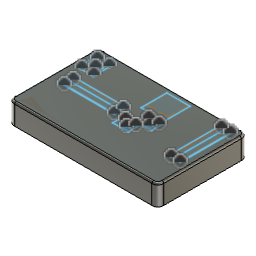
gamepad-g43 (Autodesk Fusion 360 design; units mm, degrees)
Autodesk Fusion 360 part; units mm, degrees
sketch "Sketch1" plane through (0, 0, 0) normal (0, 0, 1) x (1, 0, 0)
  line L0 (-125, 75) -> (125, 75)
  line L1 (125, 75) -> (125, -75)
  line L2 (125, -75) -> (-125, -75)
  line L3 (-125, -75) -> (-125, 75)
  line L4 (-125, 75) -> (125, -75) construction
  dimension "d1" = 250
  dimension "d2" = 150
  constraint horizontal L0
  constraint vertical L1
  constraint horizontal L2
  constraint vertical L3
  constraint midpoint origin L4
  measures "d1" distance of L0.start L0.end
  measures "d2" distance of L0.start L2.end
extrude "Extrude1" add sketch "Sketch1" along normal blind 35
sketch "Sketch3" plane through (0, 0, 0) normal (0, 0, 1) x (1, 0, 0)
  line L0 (-125, -75) -> (125, -75)
  line L1 (125, -75) -> (125, 75)
  line L2 (125, 75) -> (-125, 75)
  line L3 (-125, 75) -> (-125, -75)
  line L4 (-122, 72) -> (122, 72)
  line L5 (122, 72) -> (122, -70)
  line L6 (122, -70) -> (-122, -70)
  line L7 (-122, -70) -> (-122, 72)
  dimension "d7" = 3
  dimension "d8" = 5
  dimension "d9" = 3
  dimension "d10" = 3
  constraint horizontal L4
  constraint vertical L5
  constraint horizontal L6
  constraint vertical L7
  measures "d7" distance of L2 L4
  measures "d8" distance of L0 L6
  measures "d9" distance of L3 L7
  measures "d10" distance of L1 L5
extrude "Extrude2" cut sketch "Sketch3" along normal blind 32 contours L4 L5 L6 L7
fillet "Fillet1" radius 3 4 edges at (125, 0, 35) (0, 75, 35) (-125, 0, 35) (0, -75, 35)
fillet "Fillet1" radius 10 curvature continuous 4 edges at (-125, -75, 17.5) (-125, 75, 17.5) (125, 75, 17.5) (125, -75, 17.5)
fillet "Fillet1" radius 8 curvature continuous 4 edges at (-122, -70, 16) (-122, 72, 16) (122, -70, 16) (122, 72, 16)
sketch "joystick" plane through (0, 0, 35) normal (0, 0, 1) x (-1, 0, 0)
  spline S0 degree 3 poles (-122, 65) (-122, 65.1579) (-122, 65.3156) (-121.9955, 66.0449) (-121.98, 66.6191) (-121.8006, 67.7625) (-121.6245, 68.3289) (-120.9937, 69.5435) (-120.4833, 70.1576) (-119.6074, 70.8914) (-119.3113, 71.0984) (-118.6838, 71.4499) (-118.3524, 71.5936) (-117.5261, 71.8524) (-117.0214, 71.9295) (-116.0107, 72.0014) (-115.5063, 72) (-115, 72) knots -1.149011 -1.149011 -1.149011 -1.149011 -1.101651 -1.101651 -0.930068 -0.930068 -0.754427 -0.754427 -0.519484 -0.519484 -0.411628 -0.411628 -0.303772 -0.303772 -0.151886 -0.151886 0 0 0 0
  line L0 (-122, 65) -> (-122, -65)
  spline S1 degree 3 poles (-115, -72) (-115.1579, -72) (-115.3156, -72) (-116.0449, -71.9955) (-116.6191, -71.98) (-117.7625, -71.8006) (-118.3289, -71.6245) (-119.5435, -70.9937) (-120.1576, -70.4833) (-120.8914, -69.6074) (-121.0984, -69.3113) (-121.4499, -68.6838) (-121.5936, -68.3524) (-121.8524, -67.5261) (-121.9295, -67.0214) (-122.0014, -66.0107) (-122, -65.5063) (-122, -65) knots -1.149011 -1.149011 -1.149011 -1.149011 -1.101651 -1.101651 -0.930068 -0.930068 -0.754427 -0.754427 -0.519484 -0.519484 -0.411628 -0.411628 -0.303772 -0.303772 -0.151886 -0.151886 0 0 0 0
  line L1 (-115, -72) -> (115, -72)
  spline S2 degree 3 poles (122, -65) (122, -65.1579) (122, -65.3156) (121.9955, -66.0449) (121.98, -66.6191) (121.8006, -67.7625) (121.6245, -68.3289) (120.9937, -69.5435) (120.4833, -70.1576) (119.6074, -70.8914) (119.3113, -71.0984) (118.6838, -71.4499) (118.3524, -71.5936) (117.5261, -71.8524) (117.0214, -71.9295) (116.0107, -72.0014) (115.5063, -72) (115, -72) knots -1.149011 -1.149011 -1.149011 -1.149011 -1.101651 -1.101651 -0.930068 -0.930068 -0.754427 -0.754427 -0.519484 -0.519484 -0.411628 -0.411628 -0.303772 -0.303772 -0.151886 -0.151886 0 0 0 0
  line L2 (122, -65) -> (122, 65)
  spline S3 degree 3 poles (115, 72) (115.1579, 72) (115.3156, 72) (116.0449, 71.9955) (116.6191, 71.98) (117.7625, 71.8006) (118.3289, 71.6245) (119.5435, 70.9937) (120.1576, 70.4833) (120.8914, 69.6074) (121.0984, 69.3113) (121.4499, 68.6838) (121.5936, 68.3524) (121.8524, 67.5261) (121.9295, 67.0214) (122.0014, 66.0107) (122, 65.5063) (122, 65) knots -1.149011 -1.149011 -1.149011 -1.149011 -1.101651 -1.101651 -0.930068 -0.930068 -0.754427 -0.754427 -0.519484 -0.519484 -0.411628 -0.411628 -0.303772 -0.303772 -0.151886 -0.151886 0 0 0 0
  line L3 (115, 72) -> (-115, 72)
  line L4 (112.7507, -62.5002) -> (86.7507, -62.5002)
  line L5 (86.7507, -62.5002) -> (86.7507, -28.5002)
  line L6 (86.7507, -28.5002) -> (112.7507, -28.5002)
  line L7 (112.7507, -28.5002) -> (112.7507, -62.5002)
  line L8 (109.7507, -58.5002) -> (89.7507, -58.5002) construction
  line L9 (89.7507, -58.5002) -> (89.7507, -32.5002) construction
  line L10 (89.7507, -32.5002) -> (109.7507, -32.5002) construction
  line L11 (109.7507, -32.5002) -> (109.7507, -58.5002) construction
  line L12 (99.7507, -58.5002) -> (99.7507, -62.5002) construction
  line L13 (89.7507, -45.5002) -> (86.7507, -45.5002) construction
  line L14 (109.7507, -45.5002) -> (112.7507, -45.5002) construction
  circle A0 centre (89.7507, -58.5002) radius 1.5
  circle A1 centre (109.7507, -58.5002) radius 1.5
  circle A2 centre (109.7507, -32.5002) radius 1.5
  circle A3 centre (89.7507, -32.5002) radius 1.5
  line L15 (99.7507, -62.5002) -> (99.7507, -45.5002) construction
  circle A4 centre (99.7507, -45.5002) radius 10
  dimension "d19" = 26
  dimension "d20" = 34
  dimension "d21" = 20
  dimension "d22" = 26
  dimension "d23" = 4
  dimension "d24" = 3
  dimension "d25" = 3
  dimension "d26" = 3
  dimension "d27" = 3
  dimension "d28" = 17
  dimension "d29" = 20
  constraint horizontal L4
  constraint vertical L5
  constraint horizontal L6
  constraint vertical L7
  constraint horizontal L8
  constraint vertical L9
  constraint horizontal L10
  constraint vertical L11
  constraint midpoint L8 L12.start
  constraint midpoint L4 L12.end
  constraint midpoint L9 L13.start
  constraint midpoint L5 L13.end
  constraint midpoint L11 L14.start
  constraint midpoint L7 L14.end
  constraint equal L13 L14
  constraint coincident L8.end L9.start
  constraint coincident L8.start L11.end
  constraint coincident L10.end L11.start
  constraint coincident L9.end L10.start
  constraint perpendicular L4 L15
  constraint coincident L15.end A4.centre
  measures "d19" distance of L4.start L4.end
  measures "d20" distance of L4.start L6.end
  measures "d21" distance of L8.start L8.end
  measures "d22" distance of L8.start L10.end
  measures "d23" distance of L4 L8
  measures "d24" diameter of A0
  measures "d25" diameter of A1
  measures "d26" diameter of A2
  measures "d27" diameter of A3
  measures "d28" distance of L12.end L15.end
  measures "d29" diameter of A4
sketch "keyboard" plane through (0, 0, 35) normal (0, 0, 1) x (-1, 0, 0)
  line L0 (0.8213, -66.0148) -> (-38.1787, -66.0148)
  line L1 (-38.1787, -66.0148) -> (-38.1787, -23.0148)
  line L2 (-38.1787, -23.0148) -> (0.8213, -23.0148)
  line L3 (0.8213, -23.0148) -> (0.8213, -66.0148)
  line L4 (-8.6787, -25.8148) -> (-28.6787, -25.8148) construction
  line L5 (-28.6787, -25.8148) -> (-28.6787, -23.0148) construction
  line L6 (-28.6787, -23.0148) -> (-8.6787, -23.0148) construction
  line L7 (-8.6787, -23.0148) -> (-8.6787, -25.8148) construction
  line L8 (-0.1787, -65.0148) -> (-35.1787, -65.0148) construction
  line L9 (-35.1787, -65.0148) -> (-35.1787, -32.0148) construction
  line L10 (-35.1787, -32.0148) -> (-0.1787, -32.0148) construction
  line L11 (-0.1787, -32.0148) -> (-0.1787, -65.0148) construction
  dimension "d30" = 39
  dimension "d31" = 43
  dimension "d32" = 20
  dimension "d33" = 2.8
  dimension "d34" = 35
  dimension "d35" = 33
  dimension "d36" = 9
  dimension "d37" = 3
  constraint horizontal L0
  constraint vertical L1
  constraint horizontal L2
  constraint vertical L3
  constraint horizontal L4
  constraint vertical L5
  constraint horizontal L6
  constraint vertical L7
  constraint midpoint L2 L6
  constraint horizontal L8
  constraint vertical L9
  constraint horizontal L10
  constraint vertical L11
  measures "d30" distance of L0.start L0.end
  measures "d31" distance of L0.start L2.end
  measures "d32" distance of L4.start L4.end
  measures "d33" distance of L4.start L6.end
  measures "d34" distance of L8.start L8.end
  measures "d35" distance of L8.start L10.end
  measures "d36" distance of L2 L10
  measures "d37" distance of L1 L9
sketch "yaw" plane through (0, 0, 35) normal (0, 0, 1) x (-1, 0, 0)
  line L0 (102.6548, -10.7995) -> (13.6548, -10.7995)
  line L1 (13.6548, -10.7995) -> (13.6548, 9.2005)
  line L2 (13.6548, 9.2005) -> (102.6548, 9.2005)
  line L3 (102.6548, 9.2005) -> (102.6548, -10.7995)
  line L4 (100.1548, -8.2995) -> (16.1548, -8.2995) construction
  line L5 (16.1548, -8.2995) -> (16.1548, 6.7005) construction
  line L6 (16.1548, 6.7005) -> (100.1548, 6.7005) construction
  line L7 (100.1548, 6.7005) -> (100.1548, -8.2995) construction
  line L8 (58.1548, -8.2995) -> (58.1548, -10.7995) construction
  line L9 (58.1548, 6.7005) -> (58.1548, 9.2005) construction
  line L10 (16.1548, -0.7995) -> (13.6548, -0.7995) construction
  line L11 (102.6548, -0.7995) -> (100.1548, -0.7995) construction
  circle A0 centre (100.1548, -8.2995) radius 1.5
  circle A1 centre (100.1548, 6.7005) radius 1.5
  circle A2 centre (16.1548, 6.7005) radius 1.5
  circle A3 centre (16.1548, -8.2995) radius 1.5
  line L12 (96.1548, -1.7995) -> (20.1548, -1.7995)
  line L13 (20.1548, -1.7995) -> (20.1548, 8.2005)
  line L14 (20.1548, 8.2005) -> (96.1548, 8.2005)
  line L15 (96.1548, 8.2005) -> (96.1548, -1.7995)
  line L16 (20.1548, 3.2005) -> (13.6548, 3.2005) construction
  line L17 (96.1548, 3.2005) -> (102.6548, 3.2005) construction
  dimension "d38" = 89
  dimension "d39" = 20
  dimension "d40" = 84
  dimension "d41" = 15
  dimension "d42" = 3
  dimension "d43" = 3
  dimension "d44" = 3
  dimension "d45" = 3
  dimension "d46" = 76
  dimension "d47" = 10
  dimension "d48" = 1
  constraint horizontal L0
  constraint vertical L1
  constraint horizontal L2
  constraint vertical L3
  constraint horizontal L4
  constraint vertical L5
  constraint horizontal L6
  constraint vertical L7
  constraint midpoint L4 L8.start
  constraint midpoint L0 L8.end
  constraint midpoint L6 L9.start
  constraint midpoint L2 L9.end
  constraint midpoint L5 L10.start
  constraint midpoint L1 L10.end
  constraint midpoint L3 L11.start
  constraint midpoint L7 L11.end
  constraint vertical L8
  constraint horizontal L11
  constraint coincident L4.start L7.end
  constraint coincident L6.end L7.start
  constraint coincident L5.end L6.start
  constraint coincident L4.end L5.start
  constraint horizontal L12
  constraint vertical L13
  constraint horizontal L14
  constraint vertical L15
  constraint midpoint L13 L16.start
  constraint coincident L1 L16.end
  constraint perpendicular L1 L16
  constraint midpoint L15 L17.start
  constraint coincident L3 L17.end
  constraint perpendicular L3 L17
  constraint equal L16 L17
  measures "d38" distance of L0.start L0.end
  measures "d39" distance of L0.start L2.end
  measures "d40" distance of L4.start L4.end
  measures "d41" distance of L4.start L6.end
  measures "d42" diameter of A0
  measures "d43" diameter of A1
  measures "d44" diameter of A2
  measures "d45" diameter of A3
  measures "d46" distance of L12.start L12.end
  measures "d47" distance of L12.start L14.end
  measures "d48" distance of L2 L14
sketch "encoder big" plane through (0, 0, 35) normal (0, 0, 1) x (-1, 0, 0)
  line L0 (-14.7711, -17.7922) -> (-40.9711, -17.7922)
  line L1 (-40.9711, -17.7922) -> (-40.9711, 1.4078)
  line L2 (-40.9711, 1.4078) -> (-14.7711, 1.4078)
  line L3 (-14.7711, 1.4078) -> (-14.7711, -17.7922)
  line L4 (-24.1711, -12.1922) -> (-36.5711, -12.1922)
  line L5 (-36.5711, -12.1922) -> (-36.5711, -0.3922)
  line L6 (-36.5711, -0.3922) -> (-24.1711, -0.3922)
  line L7 (-24.1711, -0.3922) -> (-24.1711, -12.1922)
  circle A0 centre (-30.3711, -6.2922) radius 3.4
  line L8 (-24.1711, -0.3922) -> (-36.5711, -12.1922) construction
  line L9 (-19.2711, -15.7922) -> (-36.4711, -15.7922) construction
  circle A1 centre (-19.2711, -15.7922) radius 1.5
  circle A2 centre (-36.4711, -15.7922) radius 1.5
  dimension "d49" = 26.2
  dimension "d50" = 19.2
  dimension "d51" = 12.4
  dimension "d52" = 11.8
  dimension "d53" = 16.8
  dimension "d54" = 17.4
  dimension "d55" = 6.8
  dimension "d57" = 2
  dimension "d58" = 4.5
  dimension "d59" = 4.5
  dimension "d60" = 3
  dimension "d61" = 3
  constraint horizontal L0
  constraint vertical L1
  constraint horizontal L2
  constraint vertical L3
  constraint horizontal L4
  constraint vertical L5
  constraint horizontal L6
  constraint vertical L7
  constraint midpoint A0.centre L8
  constraint parallel L0 L9
  constraint coincident L9.start A1.centre
  constraint coincident L9.end A2.centre
  measures "d49" distance of L0.start L0.end
  measures "d50" distance of L0.start L2.end
  measures "d51" distance of L4.start L4.end
  measures "d52" distance of L4.start L6.end
  measures "d53" distance of L1 L7
  measures "d54" distance of L0 L6
  measures "d55" diameter of A0
  measures "d57" distance of L0 L9
  measures "d58" distance of L3 L9.start
  measures "d59" distance of L1 L9.end
  measures "d60" diameter of A1
  measures "d61" diameter of A2
sketch "encoder small" plane through (0, 0, 35) normal (0, 0, 1) x (-1, 0, 0)
  line L0 (-19.076, 21.1996) -> (-6.676, 21.1996)
  circle A0 centre (-1.776, 5.7996) radius 1.5
  line L1 (2.724, 3.7996) -> (-23.476, 3.7996)
  circle A1 centre (-18.976, 5.7996) radius 1.5
  line L2 (-1.776, 5.7996) -> (-18.976, 5.7996) construction
  line L3 (-6.676, 21.1996) -> (-6.676, 9.3996)
  line L4 (-23.476, 3.7996) -> (-23.476, 22.9996)
  line L5 (-6.676, 21.1996) -> (-19.076, 9.3996) construction
  line L6 (2.724, 22.9996) -> (2.724, 3.7996)
  line L7 (-6.676, 9.3996) -> (-19.076, 9.3996)
  line L8 (-23.476, 22.9996) -> (2.724, 22.9996)
  line L9 (-19.076, 9.3996) -> (-19.076, 21.1996)
  circle A2 centre (-12.876, 15.2996) radius 3.4
  dimension "d74" = 26.2
  dimension "d75" = 19.2
  dimension "d76" = 12.4
  dimension "d77" = 11.8
  dimension "d78" = 16.8
  dimension "d79" = 17.4
  dimension "d80" = 6.8
  dimension "d81" = 2
  dimension "d82" = 4.5
  dimension "d83" = 4.5
  dimension "d84" = 3
  dimension "d85" = 3
  constraint horizontal L1
  constraint vertical L4
  constraint horizontal L8
  constraint vertical L6
  constraint horizontal L7
  constraint vertical L9
  constraint horizontal L0
  constraint vertical L3
  constraint midpoint A2.centre L5
  constraint parallel L1 L2
  constraint coincident A0.centre L2.start
  constraint coincident A1.centre L2.end
  measures "d74" distance of L1.end L1.start
  measures "d75" distance of L1.start L6.start
  measures "d76" distance of L3.end L5.end
  measures "d77" distance of L3.end L0.end
  measures "d78" distance of L3 L4
  measures "d79" distance of L0 L1
  measures "d80" diameter of A2
  measures "d81" distance of L1 L2
  measures "d82" distance of A0.centre L6
  measures "d83" distance of A1.centre L4
  measures "d84" diameter of A0
  measures "d85" diameter of A1
sketch "throttle" plane through (0, 0, 35) normal (0, 0, 1) x (-1, 0, 0)
  line L0 (-105.681, 17.5) -> (-105.681, 24) construction
  line L1 (-110.681, -58.5) -> (-110.681, 17.5)
  line L2 (-105.681, -58.5) -> (-105.681, -65) construction
  line L3 (-94.181, 21.5) -> (-94.181, -62.5) construction
  line L4 (-109.181, -20.5) -> (-111.681, -20.5) construction
  circle A0 centre (-94.181, 21.5) radius 1.5
  line L5 (-109.181, -62.5) -> (-109.181, 21.5) construction
  circle A1 centre (-109.181, -62.5) radius 1.5
  line L6 (-100.681, -58.5) -> (-110.681, -58.5)
  line L7 (-94.181, -62.5) -> (-109.181, -62.5) construction
  line L8 (-91.681, -65) -> (-111.681, -65)
  line L9 (-101.681, 24) -> (-101.681, 21.5) construction
  line L10 (-111.681, 24) -> (-91.681, 24)
  line L11 (-111.681, -65) -> (-111.681, 24)
  circle A2 centre (-94.181, -62.5) radius 1.5
  line L12 (-91.681, 24) -> (-91.681, -65)
  line L13 (-94.181, -20.5) -> (-91.681, -20.5) construction
  line L14 (-101.681, -62.5) -> (-101.681, -65) construction
  line L15 (-100.681, 17.5) -> (-100.681, -58.5)
  circle A3 centre (-109.181, 21.5) radius 1.5
  line L16 (-110.681, 17.5) -> (-100.681, 17.5)
  line L17 (-109.181, 21.5) -> (-94.181, 21.5) construction
  dimension "d86" = 89
  dimension "d87" = 20
  dimension "d88" = 84
  dimension "d89" = 15
  dimension "d90" = 3
  dimension "d91" = 3
  dimension "d92" = 3
  dimension "d93" = 3
  dimension "d94" = 76
  dimension "d95" = 10
  dimension "d96" = 1
  constraint midpoint L13.start L3
  constraint midpoint L13.end L12
  constraint midpoint L4.start L5
  constraint midpoint L4.end L11
  constraint midpoint L14.start L7
  constraint midpoint L14.end L8
  constraint midpoint L9.start L10
  constraint midpoint L9.end L17
  constraint coincident L3.start A0.centre
  constraint coincident L5.end A3.centre
  constraint coincident L5.start A1.centre
  constraint coincident L3.end L7.start
  constraint midpoint L2.start L6
  constraint coincident L2.end L8
  constraint perpendicular L2 L8
  constraint midpoint L0.start L16
  constraint coincident L0.end L10
  constraint perpendicular L0 L10
  constraint equal L0 L2
  constraint horizontal L10
  constraint vertical L11
  constraint vertical L12
  constraint horizontal L8
  constraint vertical L15
  constraint horizontal L6
  constraint horizontal L16
  constraint horizontal L13
  constraint horizontal L4
  constraint equal L4 L13
  constraint horizontal L7
  constraint vertical L5
  constraint vertical L3
  measures "d86" distance of L8.start L10.end
  measures "d87" distance of L10.end L10.start
  measures "d88" distance of L3.start L3.end
  measures "d89" distance of L3.start L5.end
  measures "d90" diameter of A0
  measures "d91" diameter of A3
  measures "d92" diameter of A1
  measures "d93" diameter of A2
  measures "d94" distance of L6.start L15.start
  measures "d95" distance of L15.start L1.end
  measures "d96" distance of L1 L11
